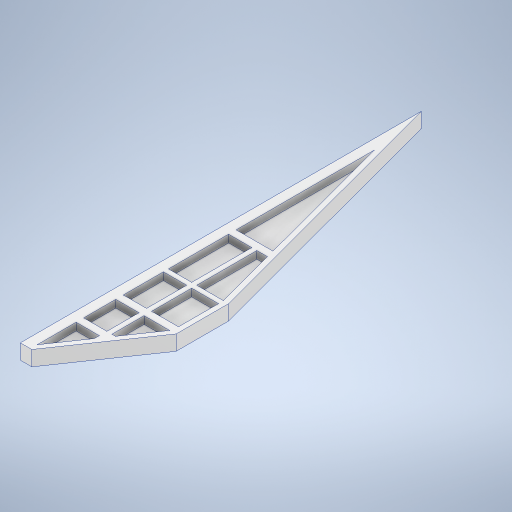
# Autodesk Inventor part: Nozki
Saved by Autodesk Inventor 2024 (Build 280153000, 153)
## iProperties
Created: 2023-08-21
Part Number: Nozki
Material: Aluminum 6061
Document SubType Name: Modeling
Designer: KirikDK
Density: 2.7 g/cm^3
Appearance: Aluminum - Flat
Mass: 2746.61 g
Surface Area: 2154.04 cm^2
Volume: 1017.26 cm^3
Author: KirikDK
Autodesk Inventor part; units mm, degrees
ref_plane "YZ Plane" through (0, 0, 0) normal (1, 0, 0) x (0, 1, 0)
ref_plane "XZ Plane" through (0, 0, 0) normal (0, 1, 0) x (-1, 0, 0)
ref_plane "XY Plane" through (0, 0, 0) normal (0, 0, 1) x (1, 0, 0)
sketch "Sketch1" plane through (0, 0, 0) normal (0, 1, 0) x (-1, 0, 0)
  line L0 (86, 229) -> (-74, 229)
  line L1 (-74, 229) -> (-74, -371)
  line L2 (-74, -371) -> (86, -371)
  line L3 (86, -371) -> (86, 229)
  line L4 (86, 229) -> (-74, 229)
  line L5 (-74, 229) -> (-74, 429)
  line L6 (-74, 429) -> (86, 429)
  line L7 (86, 429) -> (86, 229)
  line L8 (-74, 229) -> (86, -371)
  line L9 (-74, 229) -> (63.0532, 429)
  line L10 (-74, 429) -> (-54, 429)
  line L11 (-54, 429) -> (-54, -371)
  line L12 (-54, -371) -> (-74, -371)
  line L13 (-74, -371) -> (-74, 429)
  point P0 (0, 0)
  point P1 (-54, 258.1857)
  point P2 (-54, 154)
  dimension "d0" = 600
  dimension "d1" = 200
  dimension "d2" = 160
  dimension "d3" = 20
  constraints: 28 end point, 6 parallel, 3 horizontal, 3 perpendicular, 2 point on line
  measures "d0" distance of L2.end L0.start
  measures "d1" distance of L6.end L0.start
  measures "d2" distance of L0.start L0.end
  measures "d3" distance between parallel lines of L1 L11
extrude "Extrusion1" add sketch "Sketch1" along normal blind 30 contours L3 L8 L11 L0 | L0 L11 L9 L6 L7
sketch "Sketch2" plane through (0, 30, 0) normal (0, 1, 0) x (1, 0, 0)
  line L0 (75.5798, -163.6757) -> (-122, -163.6757)
  line L1 (-122, -163.6757) -> (-122, -153.6757)
  line L2 (-122, -153.6757) -> (75.5798, -153.6757)
  line L3 (75.5798, -153.6757) -> (75.5798, -163.6757)
  line L4 (143.751, -33.6757) -> (-97.1737, -33.6757)
  line L5 (-97.1737, -33.6757) -> (-97.1737, -18.6757)
  line L6 (-97.1737, -18.6757) -> (143.751, -18.6757)
  line L7 (143.751, -18.6757) -> (143.751, -33.6757)
  line L8 (152.9485, -258.6757) -> (-87.9762, -258.6757)
  line L9 (-87.9762, -258.6757) -> (-87.9762, -243.6757)
  line L10 (-87.9762, -243.6757) -> (152.9485, -243.6757)
  line L11 (152.9485, -243.6757) -> (152.9485, -258.6757)
  line L12 (-86, -429) -> (-63.0532, -429) projected
  line L13 (-63.0532, -429) -> (54, -258.1857) projected
  line L14 (54, -258.1857) -> (54, -154) projected
  line L15 (54, -154) -> (-86, 371) projected
  line L16 (-86, 371) -> (-86, -429) projected
  line L17 (-76, -419) -> (-68.3232, -419)
  line L18 (-68.3232, -419) -> (44, -255.0882)
  line L19 (44, -255.0882) -> (44, -155.3104)
  line L20 (44, -155.3104) -> (-76, 294.6896)
  line L21 (-76, 294.6896) -> (-76, -419)
  line L22 (38.103, -337.8179) -> (-236.6655, -337.8179)
  line L23 (-236.6655, -337.8179) -> (-236.6655, -322.8179)
  line L24 (-236.6655, -322.8179) -> (38.103, -322.8179)
  line L25 (38.103, -322.8179) -> (38.103, -337.8179)
  line L26 (-19.6002, -33.6757) -> (-9.6002, -33.6757)
  line L27 (-9.6002, -33.6757) -> (-9.6002, -433)
  line L28 (-9.6002, -433) -> (-19.6002, -433)
  line L29 (-19.6002, -433) -> (-19.6002, -33.6757)
  line L30 (-76, -419) -> (-66, -419)
  line L31 (-66, -419) -> (-66, 295.0501)
  line L32 (-66, 295.0501) -> (-76, 295.0501)
  line L33 (-76, 295.0501) -> (-76, -419)
  point P0 (0, 0)
  point P1 (-76, -18.6757)
  point P2 (7.5641, -18.6757)
  point P3 (-76, -33.6757)
  point P4 (-76, -153.6757)
  point P5 (44, -159.6038)
  point P6 (11.5641, -33.6757)
  point P7 (-76, -163.6757)
  point P8 (-76, -243.6757)
  point P9 (38.3772, -263.2935)
  point P10 (44, -163.6757)
  point P11 (41.5416, -258.6757)
  point P12 (-76, -258.6757)
  point P13 (-94.6892, -355.1147)
  point P14 (-104.6892, -352.0171)
  point P15 (43.5641, -153.6757)
  point P16 (44, -243.6757)
  point P17 (-86, -163.6757)
  point P18 (-86, -243.6757)
  point P19 (-86, -33.6757)
  point P20 (-86, -153.6757)
  point P21 (53.9135, -153.6757)
  point P22 (21.9135, -33.6757)
  point P23 (17.9135, -18.6757)
  point P24 (-86, -18.6757)
  point P25 (-86, -258.6757)
  point P26 (54, -163.6757)
  point P27 (-86, -337.8179)
  point P28 (-86, -322.8179)
  point P29 (54, -243.6757)
  point P30 (53.6642, -258.6757)
  point P31 (9.7098, -322.8179)
  point P32 (-0.5692, -337.8179)
  point P33 (-9.6002, -350.9967)
  point P34 (-19.6002, -365.5895)
  point P35 (-66, 257.1896)
  point P36 (-66, -18.6757)
  point P37 (-9.6002, -33.6757)
  point P38 (-9.6002, -153.6757)
  point P39 (-66, -33.6757)
  point P40 (-66, -153.6757)
  point P41 (-19.6002, -153.6757)
  point P42 (-66, -163.6757)
  point P43 (-66, -243.6757)
  point P44 (-19.6002, -243.6757)
  point P45 (-19.6002, -163.6757)
  point P46 (-9.6002, -163.6757)
  point P47 (-9.6002, -243.6757)
  point P48 (-9.6002, -258.6757)
  point P49 (-9.6002, -322.8179)
  point P50 (-2.4129, -322.8179)
  point P51 (-66, -258.6757)
  point P52 (-66, -322.8179)
  point P53 (-19.6002, -322.8179)
  point P54 (-19.6002, -258.6757)
  point P55 (-66, -337.8179)
  point P56 (-66, -415.6098)
  point P57 (-19.6002, -347.8991)
  point P58 (-19.6002, -337.8179)
  dimension "d6" = 10
  dimension "d7" = 15
  dimension "d8" = 15
  dimension "d9" = 120
  dimension "d10" = 80
  dimension "d11" = 10
  dimension "d15" = 15
  dimension "d16" = 10
  dimension "d17" = 20
  constraints: 58 end point, 12 parallel, 6 horizontal, 6 perpendicular, 1 point on line, 4 other
  measures "d6" distance of L0.end L1.end
  measures "d7" distance of L4.end L5.end
  measures "d8" distance of L8.end L9.end
  measures "d9" distance between parallel lines of L4 L2
  measures "d10" distance between parallel lines of L10 L0
  measures "d11" distance between parallel lines of L16 L21
  measures "d15" distance of L23.start L23.end
  measures "d16" distance of L27.end L28.end
  measures "d17" distance between parallel lines of L16 L31
extrude "Extrusion2" cut sketch "Sketch2" against normal blind 15 contours L19 L10 L27 L0 | L2 L27 L4 L20 | L29 L10 L31 L0 | L2 L31 L4 L29 | L8 L18 L24 L27 | L6 L31 L20 | L29 L24 L31 L8 | L29 L18 L31 L22
body "Solid1"
